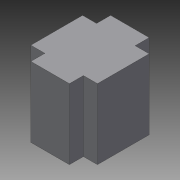
# Autodesk Inventor part: Stepper_Motor_Large
Saved by Autodesk Inventor 2015 (Build 190159000, 159)
## iProperties
Created: 2014-12-25
Part Number: Stepper_Motor_Large
Material: Generic
Document SubType Name: Modeling
Designer: Drew
Density: 1 g/cm^3
Appearance: Default
Author: Drew
Autodesk Inventor part; units mm, degrees
ref_plane "YZ Plane" through (0, 0, 0) normal (1, 0, 0) x (0, 1, 0)
ref_plane "XZ Plane" through (0, 0, 0) normal (0, 1, 0) x (-1, 0, 0)
ref_plane "XY Plane" through (0, 0, 0) normal (0, 0, 1) x (1, 0, 0)
sketch "Sketch1" plane through (0, 0, 0) normal (0, 1, 0) x (-1, 0, 0)
  line L0 (-12.0638, -14.4483) -> (12.0638, -14.4483)
  line L1 (12.0638, -14.4483) -> (12.0638, 14.4483)
  line L2 (12.0638, 14.4483) -> (-12.0638, 14.4483)
  line L3 (-12.0638, 14.4483) -> (-12.0638, -14.4483)
  line L4 (-12.0638, -14.4483) -> (12.0638, 14.4483) construction
  line L5 (12.0638, -14.4483) -> (-12.0638, 14.4483) construction
  line L6 (12.0638, 14.4483) -> (6.9838, 14.4483)
  line L7 (6.9838, 14.4483) -> (6.9838, 9.3683)
  line L8 (6.9838, 9.3683) -> (12.0638, 9.3683)
  line L9 (12.0638, 9.3683) -> (12.0638, 14.4483)
  line L10 (15.7012, 0) -> (-14.7312, 0)
  line L11 (0, 21.5613) -> (0, -24.5212)
  line L12 (12.0638, -14.4483) -> (6.9838, -14.4483)
  line L13 (6.9838, -14.4483) -> (6.9838, -9.3683)
  line L14 (6.9838, -9.3683) -> (12.0638, -9.3683)
  line L15 (12.0638, -9.3683) -> (12.0638, -14.4483)
  line L16 (-12.0638, 14.4483) -> (-6.9838, 14.4483)
  line L17 (-6.9838, 14.4483) -> (-6.9838, 9.3683)
  line L18 (-6.9838, 9.3683) -> (-12.0638, 9.3683)
  line L19 (-12.0638, 9.3683) -> (-12.0638, 14.4483)
  line L20 (-12.0638, -14.4483) -> (-6.9838, -14.4483)
  line L21 (-6.9838, -14.4483) -> (-6.9838, -9.3683)
  line L22 (-6.9838, -9.3683) -> (-12.0638, -9.3683)
  line L23 (-12.0638, -9.3683) -> (-12.0638, -14.4483)
  point P0 (0, 0)
  point P1 (0, 0)
  point P2 (0, 0)
  dimension "d0" = 28.8966
  dimension "d1" = 24.1277
  dimension "d2" = 5.08
  dimension "d3" = 5.08
  constraints: 48 end point, 9 symmetric about line, 4 midpoint, 4 parallel, 3 horizontal, 2 perpendicular, 2 point on line, 1 vertical
  measures "d0" distance of L0.end L1.end
  measures "d1" distance of L1.end L2.end
  measures "d2" distance of L18.start L18.end
  measures "d3" distance of L17.start L18.start
extrude "Extrusion1" add sketch "Sketch1" along normal blind 25.4 contours L21 L22 L3 L10 L11 L0 | L11 L10 L1 L14 L13 L0 | L3 L18 L17 L2 L11 L10 | L11 L2 L7 L8 L1 L10
equation "\"d3\" = d2"
body "Solid1"
